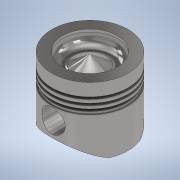
# Autodesk Inventor part: piston
Saved by Autodesk Inventor 2021 (Build 250183000, 183)
## iProperties
Created: 2020-11-23
Part Number: piston
Material: Сталь, высокопрочная, низколегированная
Document SubType Name: Modeling
Designer: panda
Mass: 1909.1 g
Surface Area: 573.952 cm^2
Volume: 243.197 cm^3
Density: 7.85 g/cm^3
Appearance: Сталь — полированная
Author: panda
Autodesk Inventor part; units mm, degrees
ref_plane "YZ Plane" through (0, 0, 0) normal (1, 0, 0) x (0, 1, 0)
ref_plane "XZ Plane" through (0, 0, 0) normal (0, 1, 0) x (-1, 0, 0)
sketch "Эскиз1" plane through (0, 0, 0) normal (0, 0, 1) x (1, 0, 0)
  line L0 (32.55, 0) -> (45.55, 0)
  line L1 (45.55, 0) -> (45.55, -80)
  line L2 (45.55, -80) -> (0, -80)
  line L3 (0, -80) -> (0, -3)
  line L4 (45.55, 0) -> (32.55, 0)
  line L5 (32.55, 0) -> (32.55, -3)
  arc A0 (22.7019, -14.7365) -> (32.55, -3) centre (22.7019, -4.7365) ccw
  line L6 (22.7019, -4.7365) -> (22.7019, -14.7365) construction
  line L7 (22.7019, -4.7365) -> (32.55, -3) construction
  line L8 (0, -3) -> (19.1679, -14.0666)
  line L9 (0, -3) -> (22.1332, -3) construction
  line L10 (21.6679, -14.7365) -> (22.7019, -14.7365)
  arc A1 (19.1679, -14.0666) -> (21.6679, -14.7365) centre (21.6679, -9.7365) ccw
  line L11 (45.55, -15) -> (39.05, -15)
  line L12 (39.05, -15) -> (39.05, -17.5)
  line L13 (39.05, -17.5) -> (45.55, -17.5)
  line L14 (45.55, -21.5) -> (39.55, -21.5)
  line L15 (39.55, -21.5) -> (39.55, -24)
  line L16 (39.55, -24) -> (45.55, -24)
  line L17 (45.55, -27.5) -> (39.55, -27.5)
  line L18 (39.55, -27.5) -> (39.55, -31)
  line L19 (39.55, -31) -> (44.05, -31)
  line L20 (44.05, -31) -> (44.05, -33.5)
  line L21 (44.05, -33.5) -> (45.55, -33.5)
  point P0 (0, 0)
  dimension "d0" = 80
  dimension "d1" = 45.55
  dimension "d2" = 13
  dimension "d3" = 3
  dimension "d5" = 10
  dimension "d6" = 30
  dimension "d7" = 3
  dimension "d8" = 5
  dimension "d9" = 180
  dimension "d10" = 2.5
  dimension "d11" = 6.5
  dimension "d12" = 2.5
  dimension "d13" = 3.5
  dimension "d14" = 4
  dimension "d15" = 15
  dimension "d17" = 2.5
  dimension "d18" = 1.5
  dimension "d20" = 6
  dimension "d21" = 6
  dimension "d22" = 3.5
  dimension "d34" = 100
  constraints: 44 end point, 11 perpendicular, 8 point on line, 5 horizontal, 4 point on circle, 2 centre point, 2 tangent, 1 equal length, 1 horizontal alignment, 1 parallel, 1 vertical, 1 vertical alignment
  measures "d0" distance of L0.end L1.end
  measures "d1" distance of point (0, 0) L0.end
  measures "d2" distance of L0.start L0.end
  measures "d3" distance of L0.start L5.end
  measures "d5" radius of A0
  measures "d6" angle of L8 L9
  measures "d7" distance from line of L3.end L0
  measures "d8" radius of A1
  measures "d9" angle of L5 L6
  measures "d10" distance of L11.end L12.end
  measures "d11" distance of L11.start L11.end
  measures "d12" distance of L14.end L15.end
  measures "d13" distance of L17.end L18.end
  measures "d14" distance of L14.start L13.end
  measures "d15" distance of L11.start L0.end
  measures "d17" distance of L19.end L20.end
  measures "d18" distance of L20.end L21.end
  measures "d20" distance of L14.start L14.end
  measures "d21" distance of L17.start L17.end
  measures "d22" distance of L17.start L16.end
  measures "d34" angle of L6 L7
revolve "Вращение1" add sketch "Эскиз1" angle 360 about axis through (0, -80, 0) along (0, 1, 0) contours L0 L1 L11 L12 L13 L14 L15 L16 L17 L18 L19 L20 L21 L2 L3 L8 A1 L10 A0 L5
sketch "Эскиз2" plane through (0, 0, 0) normal (0, 0, 1) x (1, 0, 0)
  line L0 (-39.05, -15) -> (39.05, -15) projected
  line L1 (-39.55, -27.5) -> (39.55, -27.5) projected
  arc A0 (0, -27.5) -> (-39.05, -66.55) centre (0, -66.55) ccw
  line L2 (0, -66.55) -> (-39.05, -66.55) construction
  line L3 (0, -66.55) -> (0, -27.5) construction
  line L4 (-39.05, -66.55) -> (-39.05, -88.4804)
  line L5 (-45.55, -80) -> (45.55, -80) projected
  line L6 (-39.05, -88.4804) -> (0, -88.4804)
  line L7 (0, -88.4804) -> (0, -27.5)
  point P0 (0, 0)
  dimension "d23" = 90
  constraints: 10 end point, 3 perpendicular, 2 point on circle, 2 vertical alignment, 1 centre point, 1 midpoint
  measures "d23" angle of L3 L2
revolve "Вращение2" cut sketch "Эскиз2" angle 360 about axis through (0, -66.55, 0) along (0, 1, 0)
sketch "Эскиз3" plane through (0, 0, 0) normal (0, 0, 1) x (1, 0, 0)
  circle A0 centre (0, -137.4535) radius 70.9035
  line L0 (-45.55, -80) -> (45.55, -80) projected
  line L1 (-41.55, -80) -> (41.55, -80)
  line L2 (-39.05, -66.55) -> (39.05, -66.55) projected
  point P0 (0, 0)
  dimension "d25" = 4
  constraints: 2 end point, 2 point on circle, 2 point on line, 1 centre point, 1 collinear, 1 tangent, 1 vertical alignment
  measures "d25" distance of L0.end L1.end
extrude "Выдавливание1" cut sketch "Эскиз3" along normal through all both and the other way through all
ref_plane "РабПлоскость1" through (0, 0, 39.05) normal (0, 0, 1) x (1, 0, 0)
sketch "Эскиз4" plane through (0, 0, 39.05) normal (0, 0, 1) x (1, 0, 0)
  circle A0 centre (0, -49.0033) radius 17.5467
  point P0 (0, 0)
  constraints: 1 centre point
extrude "Выдавливание2" add sketch "Эскиз4" against normal blind 20
mirror "Зеркальное отражение1" about plane through (0, 0, 0) normal (0, 0, 1) of "Выдавливание2"
sketch "Эскиз5" plane through (0, -49.0033, -19.05) normal (0, 0, 1) x (1, 0, 0)
  arc A0 (-8.1007, 15.5649) -> (8.1007, 15.5649) centre (0, 0) ccw projected
  circle A1 centre (0, 0) radius 14
  point P0 (0, 49.0033)
  dimension "d31" = 28
  constraints: 1 centre point, 1 coincident
  measures "d31" diameter of A1
extrude "Выдавливание3" cut sketch "Эскиз5" along normal through all both and the other way through all
